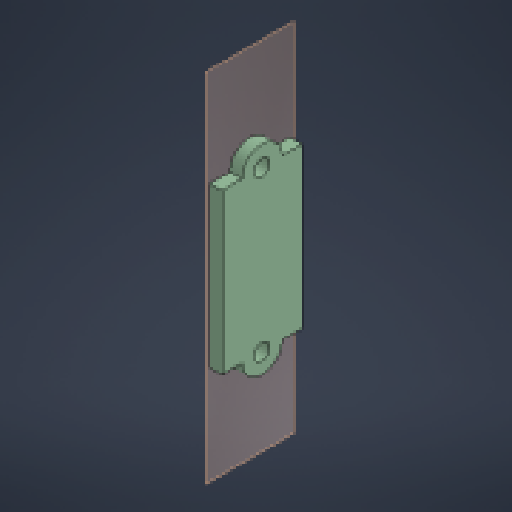
# Autodesk Inventor part: BallSensor_PCB
Saved by Autodesk Inventor 2024.2 (Build 282272000, 272)
## iProperties
Created: 2023-12-28
Part Number: BallSensor_PCB
Material: 一般
Document SubType Name: Modeling
Designer: Hanaoka
Density: 1 g/cm^3
Appearance: 既定
Author: Hanaoka
Autodesk Inventor part; units mm, degrees
ref_plane "YZ Plane" through (0, 0, 0) normal (1, 0, 0) x (0, 1, 0)
ref_plane "XZ Plane" through (0, 0, 0) normal (0, 1, 0) x (-1, 0, 0)
ref_plane "XY Plane" through (0, 0, 0) normal (0, 0, 1) x (1, 0, 0)
ref_plane "作業平面1" through (-13.5408, -19.6489, 22.9398) normal (1, 0, 0) x (0, 1, 0)
sketch "スケッチ1" plane through (-13.5408, -19.6489, 22.9398) normal (1, 0, 0) x (0, 1, 0)
  circle A0 centre (24.25, -4) radius 0.8 projected
  circle A1 centre (8.25, -4) radius 0.8 projected
  arc A2 (24.25, -6) -> (24.25, -2) centre (24.25, -4) ccw
  arc A3 (8.25, -2) -> (8.25, -6) centre (8.25, -4) ccw
  line L0 (24.25, -2) -> (24.25, 0)
  line L1 (24.25, 0) -> (8.25, 0)
  line L2 (8.25, 0) -> (8.25, -2)
  line L3 (8.25, -6) -> (8.25, -8)
  line L4 (8.25, -8) -> (24.25, -8)
  line L5 (24.25, -8) -> (24.25, -6)
  line L6 (24.25, -2) -> (24.25, -6) construction
  point P0 (19.6489, -22.9398)
  dimension "d0" = 2
  dimension "d1" = 8
  constraints: 14 end point, 4 equal length, 4 point on circle, 3 coincident, 3 perpendicular, 2 centre point, 2 parallel, 2 vertical, 1 equal radius, 1 midpoint
  measures "d0" radius of A2
  measures "d1" distance between parallel lines of L4 L1
extrude "押し出し1" add sketch "スケッチ1" along normal blind 1.2
